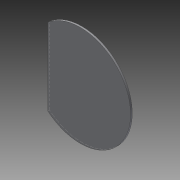
# Autodesk Inventor part: top plate
Saved by Autodesk Inventor 2015 (Build 190159000, 159)
## iProperties
Created: 2014-08-11
Part Number: top plate
Material: Generic
Document SubType Name: Modeling
Designer: karl
Density: 1 g/cm^3
Appearance: Default
Author: karl
Autodesk Inventor part; units mm, degrees
ref_plane "YZ Plane" through (0, 0, 0) normal (1, 0, 0) x (0, 1, 0)
ref_plane "XZ Plane" through (0, 0, 0) normal (0, 1, 0) x (-1, 0, 0)
ref_plane "XY Plane" through (0, 0, 0) normal (0, 0, 1) x (1, 0, 0)
sketch "Sketch1" plane through (0, 0, 0) normal (0, 1, 0) x (-1, 0, 0)
  circle A0 centre (0, 0) radius 85
  line L0 (55, 64.8074) -> (55, -64.8074)
  dimension "d0" = 170
  dimension "d1" = 55
  constraints: 2 end point, 2 point on circle, 1 centre point, 1 coincident, 1 vertical
  measures "d0" diameter of A0
  measures "d1" distance from line of point (0, 0) L0
extrude "Extrusion1" add sketch "Sketch1" along normal blind 3 contours L0 A0 picked at (8.3333, 0)
sketch "Sketch2" plane through (0, 3, 0) normal (0, 1, 0) x (1, 0, 0)
  line L0 (-27.5, -70) -> (27.5, -70)
  line L1 (27.5, -70) -> (27.5, -55)
  line L2 (27.5, -55) -> (-27.5, -55)
  line L3 (-27.5, -55) -> (-27.5, -70)
  point P0 (0, 0)
  point P1 (0, -70)
  dimension "d4" = 55
  dimension "d5" = 15
  dimension "d6" = 55
  constraints: 8 end point, 2 parallel, 1 horizontal, 1 midpoint, 1 perpendicular, 1 vertical alignment
  measures "d4" distance from line of point (0, 0) L2
  measures "d5" distance of L2.end L0.start
  measures "d6" distance between parallel lines of L1 L3
body "Solid1"
